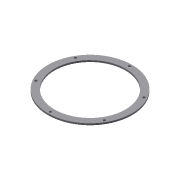
# Autodesk Inventor part: Dichtring
Saved by Autodesk Inventor 2015 (Build 190159000, 159)
## iProperties
Created: 2016-02-15
Part Number: Dichtring
Material: Generisch
Document SubType Name: Modeling
Designer: R. Demir
Density: 1 g/cm^3
Appearance: Vorgabe
Author: R. Demir
Autodesk Inventor part; units mm, degrees
ref_plane "YZ Plane" through (0, 0, 0) normal (1, 0, 0) x (0, 1, 0)
ref_plane "XZ Plane" through (0, 0, 0) normal (0, 1, 0) x (-1, 0, 0)
ref_plane "XY Plane" through (0, 0, 0) normal (0, 0, 1) x (1, 0, 0)
sketch "Skizze1" plane through (0, 0, 0) normal (0, 0, 1) x (1, 0, 0)
  circle A0 centre (0, 0) radius 43
  circle A1 centre (0, 0) radius 51
  circle A2 centre (0, 48) radius 1.5
  circle A3 centre (-41.5692, 24) radius 1.5
  circle A4 centre (-41.5692, -24) radius 1.5
  circle A5 centre (0, -48) radius 1.5
  circle A6 centre (41.5692, -24) radius 1.5
  circle A7 centre (41.5692, 24) radius 1.5
  dimension "d0" = 86
  dimension "d1" = 102
  dimension "d2" = 48
  dimension "d3" = 3
  dimension "d6" = 360
  constraints: 8 centre point, 3 coincident, 13 other
  measures "d0" diameter of A0
  measures "d1" diameter of A1
  measures "d2" distance of point (0, 48) point (0, 0)
  measures "d3" diameter of A2
extrude "Extrusion1" add sketch "Skizze1" along normal blind 2
